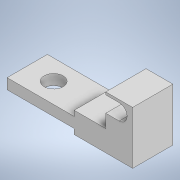
# Autodesk Inventor part: end axle
Saved by Autodesk Inventor 2020.2 (Build 242310000, 310)
## iProperties
Created: 2020-04-13
Part Number: end axle
Material: Generic
Document SubType Name: Modeling
Designer: ColinP
Density: 1 g/cm^3
Appearance: Default
Author: ColinP
Autodesk Inventor part; units mm, degrees
ref_plane "YZ Plane" through (0, 0, 0) normal (1, 0, 0) x (0, 1, 0)
ref_plane "XZ Plane" through (0, 0, 0) normal (0, 1, 0) x (-1, 0, 0)
ref_plane "XY Plane" through (0, 0, 0) normal (0, 0, 1) x (1, 0, 0)
sketch "Sketch1" plane through (0, 0, 0) normal (0, 1, 0) x (-1, 0, 0)
  line L0 (15.6447, 3.8822) -> (-8.1043, 3.8822)
  line L1 (-8.1043, 3.8822) -> (-8.1043, -3.7378)
  line L2 (-8.1043, -3.7378) -> (15.6447, -3.7378)
  line L3 (15.6447, -3.7378) -> (15.6447, 3.8822)
  point P0 (0, 0)
  dimension "d0" = 23.749
  dimension "d1" = 7.62
  constraints: 8 end point, 2 parallel, 1 horizontal, 1 perpendicular
  measures "d0" distance of L2.end L1.end
  measures "d1" distance of L1.end L0.end
extrude "Extrusion1" add sketch "Sketch1" along normal blind 1.9812
sketch "Sketch2" plane through (8.1043, 0, 3.8822) normal (1, 0, 0) x (0, 0, -1)
  line L0 (0, 0) -> (0, 1.9812) projected
  line L1 (0, 0.9906) -> (0, 2.9845)
  line L2 (0, 2.9845) -> (7.62, 2.9845)
  line L3 (7.62, 2.9845) -> (7.62, -1.0033)
  line L4 (7.62, -1.0033) -> (0, -1.0033)
  line L5 (0, -1.0033) -> (0, 2.9845)
  point P0 (3.8822, 0)
  dimension "d4" = 1.9939
  dimension "d5" = 3.9878
  constraints: 10 end point, 2 parallel, 1 collinear, 1 horizontal, 1 midpoint, 1 perpendicular
  measures "d4" distance of L1.start L1.end
  measures "d5" distance of L2.end L3.end
extrude "Extrusion2" add sketch "Sketch2" against normal blind 11.049
sketch "Sketch3" plane through (8.1043, 2.9845, 3.8822) normal (0, 1, 0) x (1, 0, 0)
  line L0 (0, 0) -> (0, 7.62) projected
  line L1 (0, 7.62) -> (-11.049, 7.62) projected
  line L2 (0, 0) -> (-5.08, 0)
  line L3 (-5.08, 0) -> (-5.08, 7.62)
  line L4 (-5.08, 7.62) -> (0, 7.62)
  line L5 (0, 7.62) -> (0, 0)
  point P0 (-8.1043, 3.8822)
  dimension "d8" = 5.08
  constraints: 8 end point, 2 parallel, 1 horizontal, 1 perpendicular, 1 point on line
  measures "d8" distance of L3.end L4.end
extrude "Extrusion3" add sketch "Sketch3" along normal blind 5.9944
sketch "Sketch4" plane through (-15.6447, 0, 3.8822) normal (0, 0, 1) x (1, 0, 0)
  line L0 (18.669, 2.9845) -> (18.669, 8.9789) projected
  line L1 (18.669, 8.9789) -> (18.669, 6.9849)
  line L2 (18.669, 6.9849) -> (21.21, 6.9849)
  circle A0 centre (21.21, 6.9849) radius 1.5
  line L3 (21.21, 8.4849) -> (18.669, 8.4849)
  line L4 (21.21, 5.4849) -> (18.669, 5.4849)
  line L5 (18.669, 8.4849) -> (18.669, 5.4849)
  point P0 (15.6447, 0)
  dimension "d11" = 1.994
  dimension "d12" = 2.541
  dimension "d13" = 3
  constraints: 10 end point, 3 point on line, 2 horizontal, 2 point on circle, 1 centre point, 1 coincident, 1 collinear, 1 parallel
  measures "d11" distance of L0.end L1.end
  measures "d12" distance of L1.end L2.end
  measures "d13" diameter of A0
extrude "Extrusion4" cut sketch "Sketch4" against normal blind 10
sketch "Sketch5" plane through (0, 1.9812, 0) normal (0, 1, 0) x (1, 0, 0)
  line L0 (-15.6447, 3.7378) -> (-15.6447, -3.8822) projected
  line L1 (-15.6447, -0.0722) -> (-10.6447, -0.0722)
  point P0 (0, 0)
  dimension "d16" = 5
  constraints: 2 end point, 1 horizontal, 1 midpoint
  measures "d16" distance of L1.start L1.end
hole "Hole1" at (-10.6447, 1.9812, 0.0722) direction (0, -1, 0) diameter 3.6 end through all clearance for "Flat Head Machine Screw" size "M3" standard "Ansi Metric M Profile"
body "Solid1"
